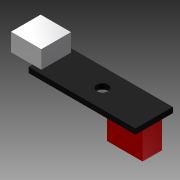
# Autodesk Inventor part: Sensor
Saved by Autodesk Inventor 2012 SP1 (Build 160190100, 190)
## iProperties
Created: 2014-02-18
Part Number: Sensor
Material: Default
Document SubType Name: Modeling
Designer: Pinkponk
Density: 1 g/cm^3
Author: Pinkponk
Autodesk Inventor part; units mm, degrees
ref_plane "YZ Plane" through (0, 0, 0) normal (1, 0, 0) x (0, 1, 0)
ref_plane "XZ Plane" through (0, 0, 0) normal (0, 1, 0) x (-1, 0, 0)
ref_plane "XY Plane" through (0, 0, 0) normal (0, 0, 1) x (1, 0, 0)
sketch "Sketch1" plane through (0, 0, 0) normal (0, 0, 1) x (1, 0, 0)
  line L0 (0, 0) -> (30, 0)
  line L1 (30, 0) -> (30, 10.5)
  line L2 (30, 10.5) -> (0, 10.5)
  line L3 (0, 10.5) -> (0, 0)
  circle A0 centre (15.5, 5.25) radius 1.6
  point P0 (0, 5.25)
  dimension "d0" = 30
  dimension "d1" = 10.5
  dimension "d2" = 3.2
  dimension "d3" = 14.5
  constraints: 8 end point, 2 parallel, 1 centre point, 1 horizontal, 1 horizontal alignment, 1 midpoint, 1 perpendicular
  measures "d0" distance of L1.end L2.end
  measures "d1" distance of L2.end L0.start
  measures "d2" diameter of A0
  measures "d3" distance from line of L1 A0.centre
extrude "Extrusion1" add sketch "Sketch1" along normal blind 1.5
sketch "Sketch2" plane through (0, 0, 1.5) normal (0, 0, 1) x (1, 0, 0)
  line L0 (0, 0) -> (0, 10.5) projected
  line L1 (30, 10.5) -> (30, 0) projected
  line L2 (-6, 9.4) -> (2.5, 9.4)
  line L3 (2.5, 9.4) -> (2.5, 1.1)
  line L4 (2.5, 1.1) -> (-6, 1.1)
  line L5 (-6, 1.1) -> (-6, 9.4)
  point P0 (-6, 5.25)
  point P1 (0, 5.25)
  dimension "d6" = 36
  dimension "d7" = 8.3
  dimension "d8" = 2.5
  constraints: 8 end point, 2 midpoint, 2 parallel, 1 horizontal, 1 horizontal alignment, 1 perpendicular
  measures "d6" distance between parallel lines of L1 L5
  measures "d7" distance between parallel lines of L4 L2
  measures "d8" distance between parallel lines of L0 L3
extrude "Extrusion2" add sketch "Sketch2" along normal blind 5
sketch "Sketch3" plane through (0, 0, 0) normal (0, 0, -1) x (-1, 0, 0)
  line L0 (-30, 0) -> (-30, 10.5) projected
  line L1 (-29.5, 8) -> (-19.5, 8)
  line L2 (-19.5, 8) -> (-19.5, 2.5)
  line L3 (-19.5, 2.5) -> (-29.5, 2.5)
  line L4 (-29.5, 2.5) -> (-29.5, 8)
  point P0 (-29.5, 5.25)
  point P1 (-30, 5.25)
  dimension "d11" = 10
  dimension "d12" = 5.5
  dimension "d13" = 0.5
  constraints: 8 end point, 2 midpoint, 2 parallel, 1 horizontal, 1 horizontal alignment, 1 perpendicular
  measures "d11" distance of L1.start L1.end
  measures "d12" distance between parallel lines of L1 L3
  measures "d13" distance between parallel lines of L0 L4
extrude "Extrusion3" add sketch "Sketch3" along normal blind 8
body "Solid1"
